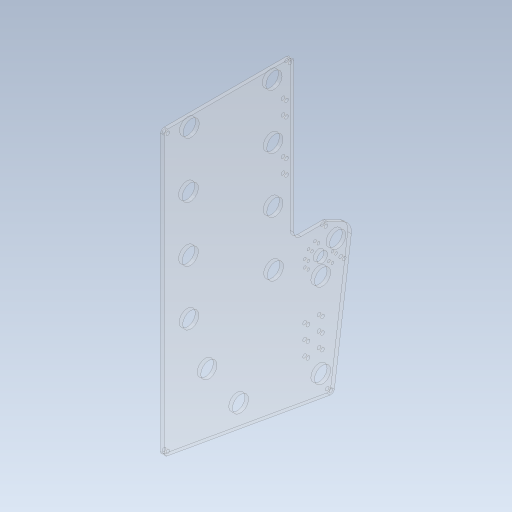
# Autodesk Inventor part: sketchers
Saved by Autodesk Inventor 2024 (Build 280153000, 153)
## iProperties
Created: 2024-07-27
Part Number: sketchers
Material: Polycarbonate, Clear
Document SubType Name: Modeling
Designer: Oscar
Density: 1.2 g/cm^3
Appearance: Polycarbonate - Clear
Mass: 1005.36 g
Surface Area: 2848.51 cm^2
Volume: 837.8 cm^3
Author: Oscar
Autodesk Inventor part; units mm, degrees
ref_plane "YZ Plane" through (0, 0, 0) normal (1, 0, 0) x (0, 1, 0)
ref_plane "XZ Plane" through (0, 0, 0) normal (0, 1, 0) x (-1, 0, 0)
ref_plane "XY Plane" through (0, 0, 0) normal (0, 0, 1) x (1, 0, 0)
sketch "Sketch1" plane through (0, 0, 0) normal (1, 0, 0) x (0, 1, 0)
  line L0 (95.25, 812.8) -> (44.45, 812.8) construction
  line L1 (44.45, 812.8) -> (44.45, 0) construction
  line L2 (44.45, 0) -> (95.25, 0) construction
  line L3 (95.25, 0) -> (95.25, 812.8) construction
  line L4 (95.25, 0) -> (44.45, 0) construction
  line L5 (44.45, 25.4) -> (95.25, 25.4) construction
  circle A0 centre (190.5, 0) radius 50.8 construction
  circle A1 centre (95.25, 279.4) radius 25.4 construction
  circle A2 centre (274.9493, 279.9916) radius 9.525
  circle A3 centre (274.9493, 279.9916) radius 25.4 construction
  circle A4 centre (274.9493, 279.9916) radius 31.75 construction
  circle A5 centre (299.4838, 286.5656) radius 2.4892
  circle A6 centre (292.9098, 297.9521) radius 2.4892
  circle A7 centre (281.5233, 304.5261) radius 2.4892
  circle A8 centre (268.3753, 304.5261) radius 2.4892
  circle A9 centre (256.9887, 297.9521) radius 2.4892
  circle A10 centre (250.4147, 286.5656) radius 2.4892 construction
  circle A11 centre (250.4147, 273.4176) radius 2.4892 construction
  circle A12 centre (256.9887, 262.0311) radius 2.4892
  circle A13 centre (268.3753, 255.4571) radius 2.4892
  circle A14 centre (281.5233, 255.4571) radius 2.4892 construction
  circle A15 centre (292.9098, 262.0311) radius 2.4892 construction
  circle A16 centre (299.4838, 273.4176) radius 2.4892
  circle A17 centre (609.6, 438.15) radius 50.8 construction
  circle A18 centre (274.9493, 279.9916) radius 30.48 construction
  circle A19 centre (587.8333, 365.125) radius 25.4 construction
  circle A20 centre (587.8333, 511.175) radius 25.4 construction
  line L6 (587.8333, 485.775) -> (587.8333, 390.525) construction
  circle A21 centre (490.3356, 512.7625) radius 14.351
  circle A22 centre (392.825, 512.7625) radius 14.351
  circle A23 centre (490.3356, 363.5375) radius 14.351
  line L7 (587.8333, 511.175) -> (490.3356, 512.7625) construction
  line L8 (587.8333, 365.125) -> (490.3356, 363.5375) construction
  circle A24 centre (490.3356, 512.7625) radius 25.4 construction
  circle A25 centre (490.3356, 363.5375) radius 25.4 construction
  line L9 (490.3356, 487.3625) -> (490.3356, 388.9375) construction
  circle A26 centre (392.825, 512.7625) radius 25.4 construction
  circle A27 centre (392.825, 363.5375) radius 25.4 construction
  circle A28 centre (392.825, 363.5375) radius 14.351
  line L10 (490.3356, 512.7625) -> (392.825, 512.7625) construction
  line L11 (490.3356, 363.5375) -> (392.825, 363.5375) construction
  line L12 (392.825, 487.3625) -> (392.825, 388.9375) construction
  circle A29 centre (295.3189, 511.8309) radius 25.4 construction
  circle A30 centre (295.3189, 362.6059) radius 25.4 construction
  circle A31 centre (203.1597, 479.9719) radius 25.4 construction
  circle A32 centre (295.3189, 511.8309) radius 14.351
  circle A33 centre (295.3189, 362.6059) radius 14.351
  circle A34 centre (203.1597, 479.9719) radius 14.351
  line L13 (392.825, 512.7625) -> (295.3189, 511.8309) construction
  line L14 (392.825, 363.5375) -> (295.3189, 362.6059) construction
  line L15 (295.3189, 486.4309) -> (295.3189, 388.0059) construction
  line L16 (295.3189, 511.8309) -> (203.1597, 479.9719) construction
  circle A35 centre (123.1487, 424.2353) radius 25.4 construction
  circle A36 centre (123.1487, 424.2353) radius 14.351
  line L17 (203.1597, 479.9719) -> (123.1487, 424.2353) construction
  circle A37 centre (95.25, 279.4) radius 14.351
  line L18 (609.6, 355.6) -> (44.45, 355.6) construction
  line L19 (44.45, 355.6) -> (44.45, 330.2) construction
  line L20 (44.45, 330.2) -> (609.6, 330.2) construction
  line L21 (609.6, 330.2) -> (609.6, 355.6) construction
  line L22 (95.25, 241.3) -> (44.45, 241.3) construction
  line L23 (44.45, 241.3) -> (44.45, 215.9) construction
  line L24 (44.45, 215.9) -> (95.25, 215.9) construction
  line L25 (95.25, 215.9) -> (95.25, 241.3) construction
  circle A38 centre (244.475, 279.4) radius 25.4 construction
  circle A39 centre (244.475, 279.4) radius 14.351
  line L26 (218.8463, 459.9947) -> (279.6322, 382.5831) construction
  circle A40 centre (274.9493, 279.9916) radius 8.89 construction
  circle A41 centre (288.401, 252.6405) radius 21.59 construction
  circle A42 centre (244.475, 279.4) radius 21.59 construction
  circle A43 centre (288.401, 252.6405) radius 14.351
  circle A44 centre (587.8333, 511.175) radius 14.351
  circle A45 centre (587.8333, 365.125) radius 14.351
  line L27 (95.25, 647.7) -> (609.6, 647.7) construction
  line L28 (609.6, 647.7) -> (609.6, 622.3) construction
  line L29 (609.6, 622.3) -> (95.25, 622.3) construction
  line L30 (95.25, 622.3) -> (95.25, 647.7) construction
  circle A46 centre (600.5333, 552.45) radius 3.2639
  circle A47 centre (600.5333, 552.45) radius 6.35 construction
  circle A48 centre (600.5333, 336.55) radius 3.2639
  circle A49 centre (600.5333, 336.55) radius 6.35 construction
  circle A50 centre (114.3, 552.45) radius 3.2639
  circle A51 centre (114.3, 552.45) radius 6.35 construction
  line L31 (595.3031, 535.4518) -> (598.6659, 546.3808) construction
  circle A52 centre (63.5, 264.8503) radius 3.2639
  circle A53 centre (63.5, 264.8503) radius 6.35 construction
  line L32 (337.9424, 330.2) -> (600.5333, 330.2)
  circle A54 centre (288.401, 252.6405) radius 24.13 construction
  circle A55 centre (244.475, 279.4) radius 24.13 construction
  line L33 (72.1591, 268.8184) -> (69.2727, 267.4957) construction
  line L34 (609.6, 342.9) -> (44.45, 342.9) construction
  circle A56 centre (288.401, 252.6405) radius 19.05 construction
  line L35 (265.0822, 266.8462) -> (267.7937, 265.1944) construction
  circle A57 centre (318.8924, 273.2978) radius 3.2639
  circle A58 centre (253.4257, 241.1003) radius 3.2639
  line L36 (95.25, 558.8) -> (44.45, 558.8) construction
  line L37 (44.45, 558.8) -> (44.45, 533.4) construction
  line L38 (44.45, 533.4) -> (95.25, 533.4) construction
  line L39 (95.25, 533.4) -> (95.25, 558.8) construction
  line L40 (114.3, 558.8) -> (600.5333, 558.8)
  line L41 (108.0468, 553.5545) -> (57.2468, 265.9549)
  line L42 (285.1949, 228.7245) -> (62.6563, 258.5566)
  circle A59 centre (318.8924, 273.2978) radius 6.35 construction
  circle A60 centre (253.4257, 241.1003) radius 6.35 construction
  arc A61 (114.3, 558.8) -> (108.0468, 553.5545) centre (114.3, 552.45) ccw
  arc A62 (57.2468, 265.9549) -> (62.6563, 258.5566) centre (63.5, 264.8503) ccw
  line L43 (312.6148, 274.2541) -> (306.3372, 275.2103) construction
  line L44 (313.6352, 269.7362) -> (308.3781, 266.1746) construction
  line L45 (259.4559, 243.09) -> (265.4861, 245.0797) construction
  line L46 (256.5005, 246.6562) -> (259.5753, 252.2121) construction
  line L47 (325.2424, 317.5) -> (325.2424, 273.2978)
  arc A63 (337.9424, 330.2) -> (325.2424, 317.5) centre (337.9424, 317.5) ccw
  line L48 (324.5494, 270.4133) -> (309.8976, 241.6792)
  arc A64 (324.5494, 270.4133) -> (325.2424, 273.2978) centre (318.8924, 273.2978) ccw
  arc A65 (285.1949, 228.7245) -> (309.8976, 241.6792) centre (288.401, 252.6405) ccw
  circle A66 centre (431.8, 342.9) radius 3.2639
  circle A67 centre (457.2, 342.9) radius 3.2639
  circle A68 centre (520.7, 342.9) radius 3.2639
  circle A69 centre (546.1, 342.9) radius 3.2639
  line L49 (606.8833, 552.45) -> (606.8833, 336.55)
  arc A70 (606.8833, 552.45) -> (600.5333, 558.8) centre (600.5333, 552.45) ccw
  arc A71 (600.5333, 330.2) -> (606.8833, 336.55) centre (600.5333, 336.55) ccw
  circle A72 centre (184.15, 304.8) radius 3.2639
  circle A73 centre (158.75, 304.8) radius 3.2639
  circle A74 centre (133.35, 304.8) radius 3.2639
  circle A75 centre (133.35, 279.4) radius 3.2639
  circle A76 centre (158.75, 279.4) radius 3.2639
  circle A77 centre (184.15, 279.4) radius 3.2639
  point P0 (0, 0)
  point P1 (274.0548, 252.2687)
  point P2 (274.7516, 257.073)
  point P3 (251.6966, 266.9984)
  point P4 (254.3358, 268.9733)
  point P5 (241.139, 234.6303)
  point P6 (100.4185, 253.4945)
  dimension "d9" = 50.8
  dimension "d14" = 50.8
  dimension "d38" = 50.8
  dimension "d53" = 50.8
  dimension "d1" = 812.8
  dimension "d2" = 44.45
  dimension "d4" = 25.4
  dimension "d5" = 101.6
  dimension "d6" = 95.25
  dimension "d8" = 50.8
  dimension "d15" = 63.5
  dimension "d21" = 19.05
  dimension "d26" = 360
  dimension "d28" = 4.9784
  dimension "d29" = 438.15
  dimension "d30" = 514.35
  dimension "d36" = 60.96
  dimension "d39" = 50.8
  dimension "d41" = 95.25
  dimension "d45" = 28.702
  dimension "d47" = 97.5106
  dimension "d48" = 98.425
  dimension "d56" = 25.4
  dimension "d73" = 50.8
  dimension "d74" = 25.4
  dimension "d75" = 215.9
  dimension "d78" = 279.4
  dimension "d80" = 149.225
  dimension "d81" = 97.5106
  dimension "d82" = 147.4978
  dimension "d83" = 17.78
  dimension "d85" = 43.18
  dimension "d92" = 330.2
  dimension "d100" = 514.35
  dimension "d107" = 25.4
  dimension "d108" = 514.35
  dimension "d109" = 266.7
  dimension "d115" = 6.5278
  dimension "d116" = 12.7
  dimension "d122" = 2.54
  dimension "d123" = 2.54
  dimension "d128" = 3.175
  dimension "d133" = 38.1
  dimension "d134" = 3.175
  dimension "d135" = 194.9958
  dimension "d136" = 6.5278
  dimension "d137" = 25.4
  dimension "d138" = 533.4
  dimension "d139" = 19.05
  dimension "d140" = 19.05
  dimension "d141" = 12.7
  dimension "d142" = 6.35
  dimension "d143" = 12.7
  dimension "d144" = 43.18
  dimension "d149" = 25.4
  dimension "d151" = 6.5278
  dimension "d157" = 25.4
  dimension "d158" = 63.5
  dimension "d159" = 12.7
  dimension "d161" = 11.4347
  dimension "d163" = 44.45
  dimension "d164" = 38.1
  dimension "d166" = 336.55
  dimension "d167" = 25.4
  dimension "d168" = 6.5278
  dimension "d169" = 25.4
  dimension "d170" = 25.4
  dimension "d173" = 25.4
  constraints: 98 end point, 68 centre point, 41 point on circle, 32 point on line, 29 equal radius, 26 coincident, 20 tangent, 13 equal length, 10 horizontal alignment, 10 parallel, 9 horizontal, 9 vertical alignment, 5 perpendicular, 4 concentric, 4 vertical, 2 midpoint, 60 other
  measures "d1" distance of L1.end L0.end
  measures "d2" distance from line of point (0, 0) L1
  measures "d4" distance of L4.end L5.start
  measures "d5" diameter of A0
  measures "d15" diameter of A4
  measures "d21" diameter of A2
  measures "d28" diameter of A16
  measures "d29" distance from line of L2 point (609.6, 438.15)
  measures "d36" diameter of A18
  measures "d39" diameter of A20
  measures "d41" distance of L6.start L6.end
  measures "d45" diameter of A21
  measures "d47" distance of L7.start L7.end
  measures "d48" distance of L9.start L9.end
  measures "d56" distance of L20.end L18.start
  measures "d73" distance of L24.end L23.end
  measures "d74" distance of L23.end L22.end
  measures "d75" distance between parallel lines of L2 L24
  measures "d78" distance from line of L2 point (95.25, 279.4)
  measures "d80" distance of point (95.25, 279.4) A38.centre
  measures "d81" distance of A38.centre A30.centre
  measures "d82" distance of point (95.25, 279.4) A35.centre
  measures "d83" diameter of A40
  measures "d85" diameter of A41
  measures "d92" distance between parallel lines of L2 L20
  measures "d107" distance between parallel lines of L29 L27
  measures "d108" distance of L28.end L29.end
  measures "d109" distance between parallel lines of L18 L29
  measures "d115" diameter of A46
  measures "d116" diameter of A47
  measures "d122" radial gap between concentric circles of A41 A54
  measures "d128" distance of L33.start L33.end
  measures "d133" diameter of A56
  measures "d134" distance of L35.start L35.end
  measures "d135" distance of A37.centre A43.centre
  measures "d136" diameter of A58
  measures "d137" distance between parallel lines of L36 L38
  measures "d138" distance between parallel lines of L2 L38
  measures "d140" distance from line of L1 A52.centre
  measures "d141" diameter of A60
  measures "d142" distance of L44.start L44.end
  measures "d143" radius of A63
  measures "d144" diameter of A42
  measures "d149" distance of A66.centre A67.centre
  measures "d151" diameter of A66
  measures "d157" distance of A69.centre A68.centre
  measures "d158" distance of A67.centre A68.centre
  measures "d159" horizontal distance of L7.start A47.centre
  measures "d161" distance of L31.start L31.end
  measures "d163" distance of L42.start point (241.139, 234.63)
  measures "d164" distance of L42.end point (100.419, 253.494)
  measures "d167" distance between parallel lines of L2 L5
  measures "d168" diameter of A72
  measures "d169" distance of A72.centre A73.centre
  measures "d170" distance of A74.centre A73.centre
  measures "d173" distance from line of A74.centre L20
extrude "Extrusion2" add sketch "Sketch1" along normal blind 6.35 contours A9 | A16 | A63 L47 A64 L48 A65 L42 A62 L41 A61 L40 A70 L49 A71 L32
body "Solid2"
